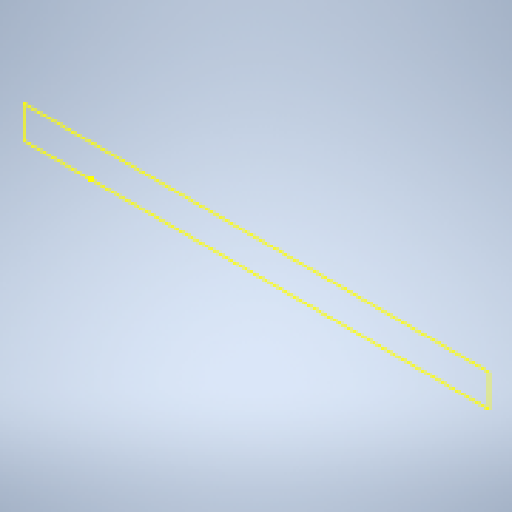
# Autodesk Inventor part: 부품72
Saved by Autodesk Inventor 2024 (Build 280153000, 153)
## iProperties
Created: 2024-09-08
Part Number: 부품72
Material: 일반
Document SubType Name: Modeling
Designer: Eungang
Density: 1 g/cm^3
Appearance: 기본값
Author: Eungang
Autodesk Inventor part; units mm, degrees
ref_plane "YZ Plane" through (0, 0, 0) normal (1, 0, 0) x (0, 1, 0)
ref_plane "XZ Plane" through (0, 0, 0) normal (0, 1, 0) x (-1, 0, 0)
ref_plane "XY Plane" through (0, 0, 0) normal (0, 0, 1) x (1, 0, 0)
sketch "스케치1" plane through (0, 0, 0) normal (0, 0, 1) x (1, 0, 0)
  line L0 (-12.2, 0) -> (71.7, 0) projected
  line L1 (71.7, 5.8) -> (71.7, 0) projected
  line L2 (-12.2, 5.8) -> (71.7, 5.8) projected
  line L3 (-12.2, 5.8) -> (-12.2, 0) projected
  line L4 (-12.2, 5.8) -> (71.7, 5.8)
  line L5 (71.7, 5.8) -> (71.7, 11.8)
  line L6 (71.7, 11.8) -> (-12.2, 11.8)
  line L7 (-12.2, 11.8) -> (-12.2, 5.8)
  line L8 (-12.2, -46.0408) -> (71.7, -46.0408) projected
  line L9 (71.7, -40.2408) -> (71.7, -46.0408) projected
  line L10 (-12.2, -40.2408) -> (71.7, -40.2408) projected
  line L11 (-12.2, -40.2408) -> (-12.2, -46.0408) projected
  line L12 (-12.2, -46.0408) -> (71.7, -46.0408)
  line L13 (71.7, -46.0408) -> (71.7, -52.0408)
  line L14 (71.7, -52.0408) -> (-12.2, -52.0408)
  line L15 (-12.2, -52.0408) -> (-12.2, -46.0408)
  line L16 (-12.2, 0) -> (71.7, 0)
  line L17 (71.7, 0) -> (71.7, -40.2408)
  line L18 (71.7, -40.2408) -> (-12.2, -40.2408)
  line L19 (-12.2, -40.2408) -> (-12.2, 0)
  point P0 (0, 0)
  dimension "d0" = 6
  dimension "d3" = 6
  constraints: 24 end point, 6 parallel, 3 horizontal, 3 perpendicular
  measures "d0" distance of L5.end L4.end
  measures "d3" distance of L12.end L13.end
extrude "돌출1" add sketch "스케치1" along normal blind 6
sketch "스케치2" plane through (0, 0, 6) normal (0, 0, 1) x (1, 0, 0)
  circle A0 centre (15, -19.9408) radius 14.2
  point P0 (0, 0)
  constraints: 1 centre point
extrude "돌출2" cut sketch "스케치2" against normal blind 6
